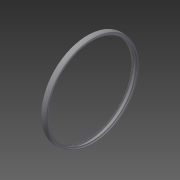
# Autodesk Inventor part: Opona_koła_tylnego
Saved by Autodesk Inventor 2015 (Build 190159000, 159)
## iProperties
Created: 2015-12-01
Part Number: Opona_koła_tylnego
Material: Aluminium AW-7020
Document SubType Name: Modeling
Designer: graaapsik
Density: 2.78 g/cm^3
Appearance: Aluminium AW-7020
Mass: 843.604 g
Surface Area: 3099.26 cm^2
Volume: 303.455 cm^3
Author: graaapsik
Autodesk Inventor part; units mm, degrees
ref_plane "YZ Plane" through (0, 0, 0) normal (1, 0, 0) x (0, 1, 0)
ref_plane "XZ Plane" through (0, 0, 0) normal (0, 1, 0) x (-1, 0, 0)
ref_plane "XY Plane" through (0, 0, 0) normal (0, 0, 1) x (1, 0, 0)
sketch "Szkic2" plane through (0, 0, 0) normal (0, 1, 0) x (-1, 0, 0)
  line L0 (-9.2588, 293.9633) -> (-12.7588, 294.9011) construction
  line L1 (-13.5, 298.6171) -> (-13.5, -298.6171) construction
  arc A0 (-13.5, 298.6171) -> (-13.9679, 299.9026) centre (-15.5, 298.6171) ccw construction
  arc A1 (-13.5, 295.8671) -> (-12.7588, 294.9011) centre (-12.5, 295.8671) ccw
  line L2 (-13.9679, 299.9026) -> (-16.0424, 302.375) construction
  line L3 (-13.5, 295.8671) -> (-13.5, 298.6171)
  line L4 (-12.7588, 294.9011) -> (-11.9213, 294.6767)
  arc A2 (-11.9213, 294.6767) -> (-11.5, 295) centre (-11.8347, 295) ccw
  arc A3 (-13.5, 298.6171) -> (-15.7502, 302.793) centre (-18.5, 298.6171) ccw
  arc A4 (-18.0284, 304.5722) -> (-17.8655, 304.4231) centre (-10.5231, 312.614) ccw
  arc A5 (-18.1647, 304.7125) -> (-18.0284, 304.5722) centre (401.6551, 712.1145) ccw
  arc A6 (0, 317.5) -> (-15, 315.5638) centre (1.7308, 245.0207) ccw
  arc A7 (-17.8655, 304.4231) -> (-15.7502, 302.793) centre (-5.8507, 317.8263) ccw
  arc A8 (-15, 315.5638) -> (-18.1647, 304.7125) centre (-13.5, 309.2392) ccw
  line L5 (0, 317.5) -> (0, 0) construction
  arc A9 (-11.5, 298.6171) -> (-14.6502, 304.4634) centre (-18.5, 298.6171) ccw
  arc A10 (-16.5305, 305.9124) -> (-14.6502, 304.4634) centre (-5.8507, 317.8263) ccw
  arc A11 (-16.6295, 306.0025) -> (-16.5305, 305.9124) centre (-10.5231, 312.614) ccw
  arc A12 (-16.7294, 306.1054) -> (-16.6295, 306.0025) centre (401.6551, 712.1145) ccw
  arc A13 (-14.5385, 313.6178) -> (-16.7294, 306.1054) centre (-13.5, 309.2392) ccw
  arc A14 (0, 315.4994) -> (-14.5385, 313.6178) centre (1.7308, 245.0207) ccw
  line L6 (-11.5, 298.6171) -> (-11.5, 295)
  line L7 (9.2588, 293.9633) -> (12.7588, 294.9011) construction
  arc A15 (13.9679, 299.9026) -> (13.5, 298.6171) centre (15.5, 298.6171) ccw construction
  arc A16 (12.7588, 294.9011) -> (13.5, 295.8671) centre (12.5, 295.8671) ccw
  line L8 (13.9679, 299.9026) -> (16.0424, 302.375) construction
  line L9 (13.5, 295.8671) -> (13.5, 298.6171)
  line L10 (12.7588, 294.9011) -> (11.9213, 294.6767)
  arc A17 (11.5, 295) -> (11.9213, 294.6767) centre (11.8347, 295) ccw
  arc A18 (15.7502, 302.793) -> (13.5, 298.6171) centre (18.5, 298.6171) ccw
  arc A19 (17.8655, 304.4231) -> (18.0284, 304.5722) centre (10.5231, 312.614) ccw
  arc A20 (18.0284, 304.5722) -> (18.1647, 304.7125) centre (-401.6551, 712.1145) ccw
  arc A21 (15, 315.5638) -> (0, 317.5) centre (-1.7308, 245.0207) ccw
  arc A22 (15.7502, 302.793) -> (17.8655, 304.4231) centre (5.8507, 317.8263) ccw
  arc A23 (18.1647, 304.7125) -> (15, 315.5638) centre (13.5, 309.2392) ccw
  arc A24 (14.6502, 304.4634) -> (11.5, 298.6171) centre (18.5, 298.6171) ccw
  arc A25 (14.6502, 304.4634) -> (16.5305, 305.9124) centre (5.8507, 317.8263) ccw
  arc A26 (16.5305, 305.9124) -> (16.6295, 306.0025) centre (10.5231, 312.614) ccw
  arc A27 (16.6295, 306.0025) -> (16.7294, 306.1054) centre (-401.6551, 712.1145) ccw
  arc A28 (16.7294, 306.1054) -> (14.5385, 313.6178) centre (13.5, 309.2392) ccw
  arc A29 (14.5385, 313.6178) -> (0, 315.4994) centre (-1.7308, 245.0207) ccw
  line L11 (11.5, 298.6171) -> (11.5, 295)
  line L12 (0, 0) -> (27.783, 0) construction
  dimension "d3" = 317.5
  dimension "d4" = 72.5
  dimension "d5" = 6.5
  dimension "d7" = 585
  dimension "d8" = 11
  dimension "d9" = 18
  dimension "d10" = 5
  dimension "d11" = 15
  dimension "d12" = 22.5
  dimension "d13" = 2
  dimension "d15" = 2
  dimension "d16" = 40
  constraints: 60 point on circle, 30 centre point, 30 symmetric about line, 24 end point, 12 tangent, 3 point on line, 2 parallel, 1 collinear, 1 perpendicular, 32 other
  measures "d3" distance of L5.start L5.end
  measures "d4" radius of A6
  measures "d5" radius of A8
  measures "d7" radius of A5
  measures "d8" radius of A4
  measures "d9" radius of A7
  measures "d10" radius of A3
  measures "d11" horizontal distance of A6.end L5.start
  measures "d12" vertical distance of L5.start A2.centre
  measures "d13" radial gap between concentric circles of A13 A8
  measures "d15" distance between parallel lines of L6 L3
revolve "Obrót1" add sketch "Szkic2" angle 360 about axis through (0, 0, 0) along (-1, 0, 0)
